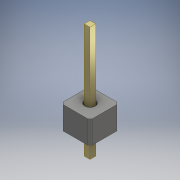
# Autodesk Inventor part: pinheader1
Saved by Autodesk Inventor 2017 (Build 210142000, 142)
## iProperties
Created: 2017-09-13
Part Number: pinheader1
Material: Generic
Document SubType Name: Modeling
Designer: erwin
Density: 1 g/cm^3
Appearance: Gold - Metal
Author: erwin
Autodesk Inventor part; units mm, degrees
ref_plane "YZ Plane" through (0, 0, 0) normal (1, 0, 0) x (0, 1, 0)
ref_plane "Work Plane1" through (0, 0, 0) normal (0, 0, 1) x (1, 0, 0)
sketch "Sketch1" plane through (0, 0, 0) normal (0, 0, 1) x (1, 0, 0)
  circle A0 centre (3.81, 25.4) radius 0.4572 projected
  circle A1 centre (3.81, 2.54) radius 0.4572 projected
  line L0 (4.06, 2.79) -> (3.56, 2.79)
  line L1 (3.56, 2.79) -> (3.56, 2.29)
  line L2 (3.56, 2.29) -> (4.06, 2.29)
  line L3 (4.06, 2.29) -> (4.06, 2.79)
  line L4 (4.06, 2.79) -> (3.56, 2.29) construction
  line L5 (3.56, 2.79) -> (4.06, 2.29) construction
  point P0 (0, 0)
  dimension "d0" = 0.5
  dimension "d1" = 0.5
  constraints: 12 end point, 2 midpoint, 2 parallel, 1 horizontal, 1 perpendicular
  measures "d0" distance of L2.end L1.end
  measures "d1" distance of L1.end L0.end
extrude "Extrusion1" add sketch "Sketch1" along normal blind 8 and the other way blind 2 contours L3 L2 L1 L0
ref_plane "Work Plane2" through (0, 0, 0) normal (0, 0, 1) x (1, 0, 0)
sketch "Sketch2" plane through (0, 0, 0) normal (0, 0, 1) x (1, 0, 0)
  circle A0 centre (3.81, 2.54) radius 0.4572 projected
  circle A1 centre (3.81, 5.08) radius 0.4572 projected
  circle A2 centre (3.81, 7.62) radius 0.4572 projected
  line L0 (5.08, 1.27) -> (2.54, 1.27)
  line L1 (2.54, 1.27) -> (2.54, 3.81)
  line L2 (2.54, 3.81) -> (5.08, 3.81)
  line L3 (5.08, 3.81) -> (5.08, 1.27)
  line L4 (5.08, 1.27) -> (2.54, 3.81) construction
  line L5 (2.54, 1.27) -> (5.08, 3.81) construction
  point P0 (0, 0)
  dimension "d6" = 2.54
  dimension "d7" = 2.54
  constraints: 12 end point, 2 midpoint, 2 parallel, 1 horizontal, 1 perpendicular
  measures "d6" distance of L1.end L2.end
  measures "d7" distance of L0.end L1.end
extrude "Extrusion2" add sketch "Sketch2" along normal blind 2 separate body contours L0 L1 L2 L3
chamfer "Chamfer1" distance 0.2 angle 45 4 edges at (2.54, 3.81, 1) (5.08, 3.81, 1) (2.54, 1.27, 1) (5.08, 1.27, 1)
body "Solid1"
body "Solid2"
